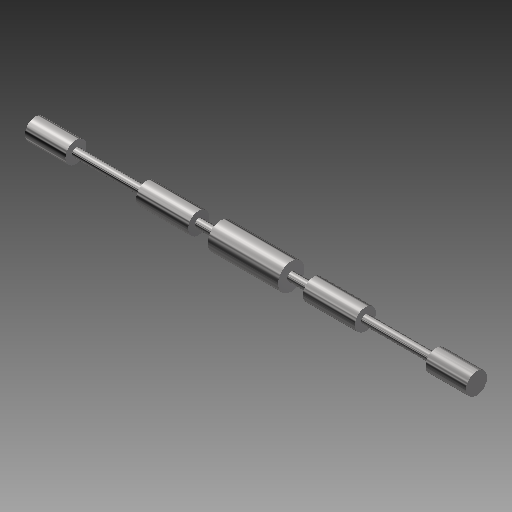
# Autodesk Inventor part: 402-03
Saved by Autodesk Inventor 2019 (Build 230136000, 136)
## iProperties
Company: Autodesk Inc.
Created: 2017-06-27
Part Number: 402-03
Material: Steel, Mild
Document SubType Name: Modeling
Designer: Autodesk Inc.
Mass: 0.163624 g
Surface Area: 0.854017 cm^2
Volume: 0.0208438 cm^3
Density: 7.85 g/cm^3
Appearance: Semi-Polished
Author: Inventor
Autodesk Inventor part; units mm, degrees
ref_plane "YZ Plane" through (0, 0, 0) normal (1, 0, 0) x (0, 1, 0)
ref_plane "XZ Plane" through (0, 0, 0) normal (0, 1, 0) x (-1, 0, 0)
ref_plane "XY Plane" through (0, 0, 0) normal (0, 0, 1) x (1, 0, 0)
sketch "Sketch1" plane through (0, 0, 0) normal (0, 0, 1) x (1, 0, 0)
  line L0 (-12.5, 0) -> (-10.2, 0)
  line L1 (-10.2, 0) -> (-10.2, 0.6)
  line L2 (-10.2, 0.6) -> (-12.5, 0.6)
  line L3 (-12.5, 0.6) -> (-12.5, 0)
  line L4 (-10.2, 0) -> (-6.2, 0)
  line L5 (-6.2, 0) -> (-6.2, 0.24)
  line L6 (-6.2, 0.24) -> (-10.2, 0.24)
  line L7 (-10.2, 0.24) -> (-10.2, 0)
  line L8 (-6.2, 0) -> (-3.25, 0)
  line L9 (-3.25, 0) -> (-3.25, 0.6)
  line L10 (-3.25, 0.6) -> (-6.2, 0.6)
  line L11 (-6.2, 0.6) -> (-6.2, 0)
  line L12 (-3.25, 0) -> (-2, 0)
  line L13 (-2, 0) -> (-2, 0.24)
  line L14 (-2, 0.24) -> (-3.25, 0.24)
  line L15 (-3.25, 0.24) -> (-3.25, 0)
  line L16 (-2, 0) -> (2, 0)
  line L17 (2, 0) -> (2, 0.75)
  line L18 (2, 0.75) -> (-2, 0.75)
  line L19 (-2, 0.75) -> (-2, 0)
  line L20 (2, 0) -> (3.25, 0)
  line L21 (3.25, 0) -> (3.25, 0.24)
  line L22 (3.25, 0.24) -> (2, 0.24)
  line L23 (2, 0.24) -> (2, 0)
  line L24 (3.25, 0) -> (6.2, 0)
  line L25 (6.2, 0) -> (6.2, 0.6)
  line L26 (6.2, 0.6) -> (3.25, 0.6)
  line L27 (3.25, 0.6) -> (3.25, 0)
  line L28 (6.2, 0) -> (10.2, 0)
  line L29 (10.2, 0) -> (10.2, 0.24)
  line L30 (10.2, 0.24) -> (6.2, 0.24)
  line L31 (6.2, 0.24) -> (6.2, 0)
  line L32 (10.2, 0) -> (12.5, 0)
  line L33 (12.5, 0) -> (12.5, 0.6)
  line L34 (12.5, 0.6) -> (10.2, 0.6)
  line L35 (10.2, 0.6) -> (10.2, 0)
  point P0 (0, 0)
  point P1 (0, 0)
  dimension "d0" = 2.3
  dimension "d1" = 6.3
  dimension "d2" = 9.25
  dimension "d3" = 10.5
  dimension "d8" = 25
  dimension "d9" = 0.48
  dimension "d10" = 1.2
  dimension "d11" = 1.5
  constraints: 72 end point, 18 parallel, 10 collinear, 9 horizontal, 9 perpendicular, 1 coincident, 1 midpoint
  measures "d0" distance between parallel lines of L1 L3
  measures "d1" distance between parallel lines of L11 L3
  measures "d2" distance between parallel lines of L9 L3
  measures "d3" distance between parallel lines of L19 L3
  measures "d8" distance between parallel lines of L33 L3
  measures "d9" diameter of L30 L32
  measures "d10" diameter of L34 L32
  measures "d11" diameter of L18 L32
revolve "Revolution1" add sketch "Sketch1" angle 360 about axis through (-6.2, 0, 0) along (1, 0, 0)
body "Solid1"
